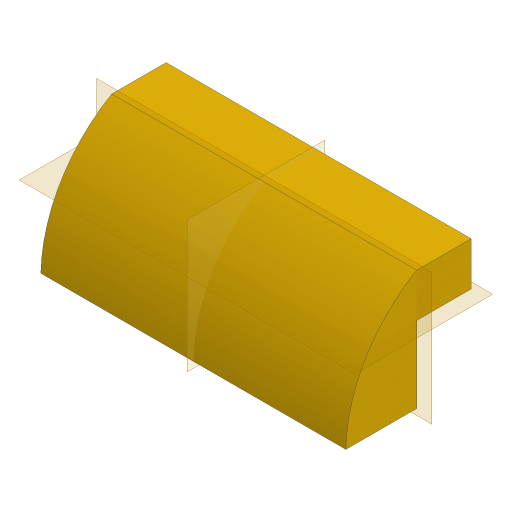
# Autodesk Inventor part: Крышка
Saved by Autodesk Inventor 2023.2 (Build 272271030, 271C)
## iProperties
Created: 2025-04-26
Part Number: Крышка
Material: Типовые
Document SubType Name: Modeling
Designer: Олег Коноваленко
Density: 1 g/cm^3
Appearance: По умолчанию
Author: Олег Коноваленко
Autodesk Inventor part; units mm, degrees
sketch "Эскиз1" plane through (0, 0, 0) normal (1, 0, 0) x (0, 1, 0)
  line L0 (-70, 65) -> (-70, 0)
  line L1 (-70, 0) -> (0, 0)
  line L2 (0, 0) -> (0, -50)
  line L3 (0, -50) -> (40, -50)
  line L4 (40, -50) -> (40, 0)
  arc A0 (40, 0) -> (-70, 65) centre (-72.5983, -64.974) ccw
  line L5 (0, 108.3305) -> (0, -93.8581) construction
  line L6 (-96.8253, 0) -> (72.7635, 0) construction
  dimension "d0" = 65
  dimension "d1" = 70
  dimension "d2" = 40
  dimension "d3" = 50
  dimension "d4" = 50
  dimension "d5" = 130
  constraints: 10 end point, 3 perpendicular, 2 point on circle, 2 point on line, 2 vertical, 1 centre point
  measures "d0" distance of L0.start L0.end
  measures "d1" distance of L0.end L1.end
  measures "d2" distance between parallel lines of L2 L4
  measures "d3" distance of L1.end L2.end
  measures "d4" distance of L3.end L4.end
  measures "d5" radius of A0
extrude "Выдавливание1" add sketch "Эскиз1" along normal mid plane 280
sketch "Эскиз2" plane through (-140, -70, 0) normal (0, -1, 0) x (1, 0, 0)
  line L0 (250, 35) -> (30, 35)
  line L1 (30, 35) -> (30, 0)
  line L2 (30, 0) -> (250, 0)
  line L3 (250, 0) -> (250, 35)
  line L4 (0, 65) -> (280, 65) projected
  line L5 (280, 65) -> (280, 0) projected
  line L6 (0, 0) -> (0, 65) projected
  line L7 (280, 0) -> (0, 0) projected
  point P0 (140, 0)
  point P1 (140, 0)
  dimension "d8" = 30
  dimension "d9" = 30
  dimension "d10" = 30
  constraints: 8 end point, 2 midpoint, 2 parallel, 1 horizontal, 1 perpendicular
  measures "d8" distance between parallel lines of L0 L4
  measures "d9" distance between parallel lines of L5 L3
  measures "d10" distance between parallel lines of L6 L1
extrude "Выдавливание2" cut sketch "Эскиз2" against normal up to surface (70 mm away) contours L3 L2 L1 L0
